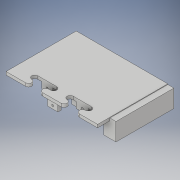
# Autodesk Inventor part: base auxiliar 2
Saved by Autodesk Inventor 2019 (Build 230136000, 136)
## iProperties
Created: 2018-08-28
Part Number: base auxiliar 2
Material: Genérico
Document SubType Name: Modeling
Designer: Albert Garangou Culebras
Density: 1 g/cm^3
Appearance: Valor por defecto
Author: Albert Garangou Culebras
Autodesk Inventor part; units mm, degrees
ref_plane "YZ Plane" through (0, 0, 0) normal (1, 0, 0) x (0, 1, 0)
ref_plane "XZ Plane" through (0, 0, 0) normal (0, 1, 0) x (-1, 0, 0)
ref_plane "XY Plane" through (0, 0, 0) normal (0, 0, 1) x (1, 0, 0)
sketch "puzzle" plane through (0, 0, 0) normal (0, 1, 0) x (-1, 0, 0)
  line L0 (0, -115) -> (-15, -115)
  line L1 (-135, -115) -> (-125, -115)
  line L2 (-135, -115) -> (-150, -115)
  line L3 (-75, -115) -> (-65, -115)
  line L4 (-75, -115) -> (-85.0002, -115)
  line L5 (-105, -135) -> (-94.9796, -135)
  line L6 (-94.9796, -135) -> (-115, -135)
  line L7 (-65, -115) -> (-60, -115)
  line L8 (-60, -125) -> (-63, -125)
  arc A0 (-60, -125) -> (-60, -115) centre (-60, -120) ccw
  arc A1 (-63, -125) -> (-63, -135) centre (-63, -130) ccw
  line L9 (-85.0002, -115) -> (-90.0002, -115)
  line L10 (-94.9796, -135) -> (-89.9796, -135)
  arc A2 (-90.0002, -115) -> (-90, -125) centre (-90.0002, -120) ccw
  arc A3 (-89.9796, -135) -> (-90, -125) centre (-89.9796, -130) ccw
  line L11 (-115, -135) -> (-120, -135)
  line L12 (-125, -115) -> (-120, -115)
  arc A4 (-120, -125) -> (-120, -115) centre (-120, -120) ccw
  arc A5 (-120, -125) -> (-120, -135) centre (-120, -130) ccw
  line L13 (0, -115) -> (-30, -115)
  line L14 (-63, -135) -> (-32.98, -135)
  line L15 (-32.98, -135) -> (-32, -135)
  line L16 (-30, -115) -> (-32, -115)
  arc A6 (-32, -115) -> (-32, -125) centre (-32, -120) ccw
  arc A7 (-32, -135) -> (-32, -125) centre (-32, -130) ccw
  line L17 (0, -115) -> (0, -230)
  line L18 (0, -230) -> (-150, -230)
  line L19 (-150, -230) -> (-150, -115)
  point P0 (0, 0)
  dimension "d22" = 5
  dimension "d23" = 5
  dimension "d24" = 5
  dimension "d25" = 5
  dimension "d26" = 5
  dimension "d76" = 115
  constraints: 40 end point, 16 point on circle, 14 horizontal, 10 tangent, 8 centre point, 3 perpendicular, 1 point on line
  measures "d22" distance of L3.end L7.end
  measures "d23" distance of L4.end L9.end
  measures "d24" distance of L5.end L10.end
  measures "d25" distance of L6.end L11.end
  measures "d26" distance of L1.end L12.end
  measures "d76" distance of L0.start L17.end
extrude "Extrusión4" add sketch "puzzle" along normal blind 5
sketch "Boceto4" plane through (0, 0, 0) normal (0, -1, 0) x (1, 0, 0)
  line L0 (0, -115) -> (0, -230) projected
  line L1 (32, -115) -> (0, -115) projected
  line L2 (0, -230) -> (10, -230)
  line L3 (150, -230) -> (0, -230) projected
  line L4 (10, -180) -> (0, -180)
  line L5 (0, -230) -> (0, -180)
  line L6 (10, -230) -> (50, -230)
  line L7 (50, -230) -> (50, -220)
  line L8 (50, -220) -> (10, -220)
  line L9 (10, -220) -> (10, -180)
  line L10 (150, -230) -> (100, -230)
  line L11 (100, -230) -> (100, -220)
  line L12 (100, -220) -> (140, -220)
  line L13 (140, -220) -> (140, -180)
  line L14 (140, -180) -> (150, -180)
  line L15 (150, -115) -> (150, -230) projected
  line L16 (150, -230) -> (150, -180)
  line L17 (70, -212.5) -> (80, -212.5)
  line L18 (80, -152.5) -> (70, -152.5)
  line L19 (45, -177.5) -> (45, -187.5)
  line L20 (105, -177.5) -> (105, -187.5)
  line L21 (83, -177.5) -> (83, -174.5)
  line L22 (83, -174.5) -> (80, -174.5)
  line L23 (80, -174.5) -> (80, -152.5)
  line L24 (83, -177.5) -> (105, -177.5)
  line L25 (80, -177.5) -> (80, -187.5)
  line L26 (80, -177.5) -> (70, -177.5)
  line L27 (67, -177.5) -> (67, -174.5)
  line L28 (67, -174.5) -> (70, -174.5)
  line L29 (67, -187.5) -> (67, -190.5)
  line L30 (67, -190.5) -> (70, -190.5)
  line L31 (67, -177.5) -> (45, -177.5)
  line L32 (67, -187.5) -> (45, -187.5)
  line L33 (70, -174.5) -> (70, -152.5)
  line L34 (70, -177.5) -> (70, -182.5)
  line L35 (70, -190.5) -> (70, -212.5)
  line L36 (80, -187.5) -> (70, -187.5)
  line L37 (70, -187.5) -> (70, -182.5)
  line L38 (80, -190.5) -> (83, -190.5)
  line L39 (83, -190.5) -> (83, -187.5)
  line L40 (80, -190.5) -> (80, -212.5)
  line L41 (83, -187.5) -> (105, -187.5)
  point P0 (0, 0)
  constraints: 76 end point, 8 perpendicular, 5 horizontal, 5 point on line, 5 vertical, 2 collinear
extrude "Extrusión5" add sketch "Boceto4" along normal blind 25
sketch "Boceto5" plane through (0, 0, 0) normal (0, -1, 0) x (1, 0, 0)
  line L0 (85, -115) -> (68, -115)
  line L1 (68, -120) -> (85, -120)
  line L2 (68, -120) -> (68, -115)
  line L3 (85, -120) -> (85, -115)
  line L4 (32, -135) -> (63, -135) projected
  line L5 (47.5, -135) -> (38.5, -135)
  line L6 (38.5, -135) -> (56.5, -135)
  line L7 (56.5, -135) -> (56.5, -140)
  line L8 (56.5, -140) -> (38.5, -140)
  line L9 (38.5, -140) -> (38.5, -135)
  line L10 (120, -135) -> (89.9796, -135) projected
  line L11 (104.9898, -135) -> (94.9898, -135)
  line L12 (94.9898, -135) -> (104.9898, -135)
  line L13 (104.9898, -135) -> (114.9898, -135)
  line L14 (114.9898, -135) -> (114.9898, -140)
  line L15 (114.9898, -140) -> (94.9898, -140)
  line L16 (94.9898, -140) -> (94.9898, -135)
  point P0 (0, 0)
  constraints: 30 end point, 4 perpendicular, 4 point on line, 3 vertical, 2 midpoint, 1 collinear, 1 horizontal
extrude "Extrusión6" add sketch "Boceto5" along normal blind 10
sketch "Boceto6" plane through (89.9796, 5, -135) normal (0, 0, 1) x (1, 0, 0)
  line L0 (10.0204, -5) -> (50.0204, -5) projected
  line L1 (25, -5) -> (15, -5)
  line L2 (25.0102, -5) -> (25.0102, -15) projected
  line L3 (25.0102, -5) -> (25.0102, -15)
  line L4 (25.0102, -15) -> (5.0102, -15) projected
  line L5 (25.0102, -15) -> (5.0102, -15)
  line L6 (15.0204, -5) -> (15.0204, -30) projected
  circle A0 centre (15.0204, -10) radius 1.6
  line L7 (-33.4796, -15) -> (-51.4796, -15) projected
  line L8 (-33.4796, -15) -> (-51.4796, -15)
  circle A1 centre (-42.4796, -10) radius 1.6
  point P0 (-89.9796, -5)
  dimension "d120" = 10
  dimension "d121" = 3.2
  dimension "d123" = 3.2
  constraints: 8 end point, 3 point on line, 2 centre point, 2 collinear, 1 vertical
  measures "d120" distance of L1.start L1.end
  measures "d121" diameter of A0
  measures "d123" diameter of A1
extrude "Extrusión7" cut sketch "Boceto6" against normal blind 10 contours A0 L6 | L6 A0 | A1
sketch "Boceto7" plane through (32, 5, -135) normal (0, 0, 1) x (1, 0, 0)
  circle A0 centre (15.5, -10) radius 1.6 projected
  circle A1 centre (15.5, -10) radius 1.6
  point P0 (-32, -5)
  constraints: 1 centre point, 1 coincident
extrude "Extrusión8" cut sketch "Boceto7" against normal blind 34
sketch "Boceto8" plane through (68, 0, -115) normal (0, 0, 1) x (1, 0, 0)
  line L0 (22.0002, 0) -> (-8, 0) projected
  line L1 (17, 0) -> (0, 0)
  line L2 (0, 0) -> (0, -10)
  line L3 (0, -10) -> (17, -10)
  line L4 (17, -10) -> (17, 0)
  circle A0 centre (8.5, -5) radius 1.6
  point P0 (-68, 0)
  dimension "d128" = 3.2
  constraints: 8 end point, 2 parallel, 1 centre point, 1 horizontal, 1 perpendicular, 1 point on line
  measures "d128" diameter of A0
extrude "Extrusión9" cut sketch "Boceto8" against normal blind 5 contours A0
sketch "Boceto9" plane through (150, 0, -115) normal (1, 0, 0) x (0, 0, -1)
  line L0 (115, 5) -> (115, -25) projected
  line L1 (20, 0) -> (10, 0) projected
  line L2 (115, 0) -> (20, 0)
  line L3 (20, 0) -> (20, -25)
  line L4 (115, -25) -> (65, -25) projected
  line L5 (20, -25) -> (115, -25)
  line L6 (115, -25) -> (115, 0)
  line L7 (115, 5) -> (115, -25) projected
  point P0 (-115, 0)
  constraints: 8 end point, 2 collinear, 1 horizontal, 1 perpendicular, 1 point on line
sketch "Boceto10" plane through (140, 0, -180) normal (0, 0, 1) x (1, 0, 0)
  line L0 (0, 0) -> (0, -25) projected
  line L1 (10, 5) -> (10, -25) projected
  line L2 (0, 0) -> (10, 0)
  line L3 (10, 0) -> (10, -25)
  line L4 (10, -25) -> (0, -25)
  line L5 (0, -25) -> (0, 0)
  point P0 (-140, 0)
  constraints: 8 end point, 2 parallel, 1 horizontal, 1 perpendicular
extrude "Extrusión10" add sketch "Boceto10" along normal blind 45
extrude "Extrusión11" add sketch "Boceto9" along normal blind 10
sketch "Boceto12" plane through (150, 0, -135) normal (0, 1, 0) x (1, 0, 0)
  line L0 (0, 0) -> (0, 95) projected
  line L1 (0, 0) -> (10, 0)
  line L2 (10, 0) -> (10, 95)
  line L3 (10, 95) -> (0, 95)
  line L4 (0, 95) -> (0, 0)
  point P0 (-150, -135)
  constraints: 8 end point, 2 parallel, 1 horizontal, 1 perpendicular
extrude "Extrusión12" add sketch "Boceto12" along normal blind 4
